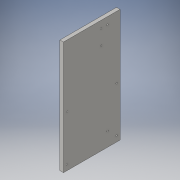
# Autodesk Inventor part: LiftPlate
Saved by Autodesk Inventor 2016 (Build 200138000, 138)
## iProperties
Created: 2017-03-04
Part Number: LiftPlate
Material: Generic
Document SubType Name: Modeling
Designer: RoboticsUser
Density: 1 g/cm^3
Appearance: Default
Author: RoboticsUser
Autodesk Inventor part; units mm, degrees
ref_plane "YZ Plane" through (0, 0, 0) normal (1, 0, 0) x (0, 1, 0)
ref_plane "XZ Plane" through (0, 0, 0) normal (0, 1, 0) x (-1, 0, 0)
ref_plane "XY Plane" through (0, 0, 0) normal (0, 0, 1) x (1, 0, 0)
sketch "Sketch1" plane through (0, 0, 0) normal (1, 0, 0) x (0, 1, 0)
  line L0 (0, 0) -> (203.2, 0)
  line L1 (203.2, 0) -> (203.2, -101.6)
  line L2 (203.2, -101.6) -> (0, -101.6)
  line L3 (0, -101.6) -> (0, 0)
  dimension "d0" = 203.2
  dimension "d1" = 101.6
  constraints: 8 end point, 2 parallel, 1 horizontal, 1 perpendicular
  measures "d0" distance of L1.end L2.end
  measures "d1" distance of L0.end L1.end
extrude "Extrusion1" add sketch "Sketch1" along normal blind 6.35
sketch "Sketch2" plane through (6.35, 0, 0) normal (1, 0, 0) x (0, 0, -1)
  line L0 (0, 0) -> (101.6, 0) projected
  line L1 (0, 203.2) -> (0, 0) projected
  line L2 (101.6, 0) -> (101.6, 203.2) projected
  line L3 (101.6, 203.2) -> (0, 203.2) projected
  point P0 (78.994, 25.4)
  point P1 (78.994, 190.5)
  dimension "d4" = 25.4
  dimension "d5" = 78.994
  dimension "d6" = 12.7
  dimension "d7" = 78.994
  measures "d4" distance from line of L0 point (78.994, 25.4)
  measures "d5" distance from line of L1 point (78.994, 25.4)
  measures "d6" distance from line of L3 point (78.994, 190.5)
  measures "d7" distance from line of L1 point (78.994, 190.5)
hole "Hole1" at (6.35, 25.4, -78.994) at (6.35, 190.5, -78.994) direction (-1, 0, 0) diameter 2.6 end through all
sketch "Sketch3" plane through (6.35, 0, 0) normal (1, 0, 0) x (0, 0, -1)
  line L0 (0, 203.2) -> (0, 0) projected
  line L1 (0, 0) -> (101.6, 0) projected
  line L2 (101.6, 0) -> (101.6, 203.2) projected
  line L3 (101.6, 203.2) -> (0, 203.2) projected
  point P0 (6.35, 10)
  point P1 (95.25, 10)
  point P2 (6.35, 91.6)
  point P3 (95.25, 91.6)
  dimension "d15" = 10
  dimension "d16" = 10
  dimension "d17" = 6.35
  dimension "d18" = 6.35
  dimension "d19" = 91.6
  dimension "d20" = 6.35
  dimension "d21" = 6.35
  dimension "d22" = 91.6
  measures "d15" distance from line of L1 point (6.35, 10)
  measures "d16" distance from line of L1 point (95.25, 10)
  measures "d17" distance from line of L0 point (6.35, 10)
  measures "d18" distance from line of L2 point (95.25, 10)
  measures "d19" distance from line of L1 point (6.35, 91.6)
  measures "d20" distance from line of L0 point (6.35, 91.6)
  measures "d21" distance from line of L2 point (95.25, 91.6)
  measures "d22" distance from line of L1 point (95.25, 91.6)
hole "Hole2" at (6.35, 10, -6.35) at (6.35, 10, -95.25) at (6.35, 91.6, -6.35) at (6.35, 91.6, -95.25) direction (-1, 0, 0) diameter 2.6 end through all
sketch "Sketch4" plane through (6.35, 0, 0) normal (1, 0, 0) x (0, 0, -1)
  line L0 (101.6, 203.2) -> (0, 203.2) projected
  line L1 (0, 203.2) -> (0, 0) projected
  line L2 (101.6, 0) -> (101.6, 203.2) projected
  line L3 (0, 0) -> (101.6, 0) projected
  circle A0 centre (78.994, 190.5) radius 1.3 projected
  point P0 (67.3608, 190.5)
  point P1 (67.3608, 163.5506)
  dimension "d30" = 12.7
  dimension "d32" = 26.9494
  dimension "d41" = 67.3608
  dimension "d42" = 67.3608
  measures "d30" distance from line of point (67.361, 190.5) L0
  measures "d32" distance of point (67.361, 163.551) point (67.361, 190.5)
  measures "d41" distance from line of L1 point (67.361, 190.5)
  measures "d42" distance from line of L1 point (67.361, 163.551)
hole "Hole3" at (6.35, 190.5, -67.3608) at (6.35, 163.5506, -67.3608) direction (-1, 0, 0) diameter 2.7781 end through all
body "Solid1"
